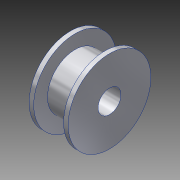
# Autodesk Inventor part: XY_Wheel-SquareBar-Rev3
Saved by Autodesk Inventor 2015 (Build 190159000, 159)
## iProperties
Created: 2017-01-08
Part Number: XY_Wheel-SquareBar-Rev3
Material: Aluminum 6061
Document SubType Name: Modeling
Designer: Guy
Density: 2.7 g/cm^3
Appearance: Aluminum - Flat
Mass: 2.90837 g
Surface Area: 12.4407 cm^2
Volume: 1.07717 cm^3
Author: Guy
Autodesk Inventor part; units mm, degrees
ref_plane "YZ Plane" through (0, 0, 0) normal (1, 0, 0) x (0, 1, 0)
ref_plane "XZ Plane" through (0, 0, 0) normal (0, 1, 0) x (-1, 0, 0)
ref_plane "XY Plane" through (0, 0, 0) normal (0, 0, 1) x (1, 0, 0)
sketch "Sketch1" plane through (0, 0, 0) normal (0, 0, 1) x (1, 0, 0)
  line L0 (0, 0) -> (0, 9)
  line L1 (0, 9) -> (1, 9)
  line L2 (1, 9) -> (1, 6)
  line L3 (1, 6) -> (7.5, 6)
  line L4 (7.5, 6) -> (7.5, 9)
  line L5 (7.5, 9) -> (8.5, 9)
  line L6 (8.5, 9) -> (8.5, 0)
  line L7 (8.5, 0) -> (0, 0)
  dimension "d0" = 8.5
  dimension "d1" = 9
  dimension "d2" = 6.5
  dimension "d3" = 6
  dimension "d9" = 1
  constraints: 16 end point, 6 perpendicular, 2 point on line, 1 vertical
  measures "d0" distance between parallel lines of L0 L6
  measures "d1" distance between parallel lines of L7 L1
  measures "d2" distance between parallel lines of L2 L4
  measures "d3" distance between parallel lines of L7 L3
  measures "d9" distance between parallel lines of L0 L2
revolve "Revolution1" add sketch "Sketch1" angle 360 about axis through (8.5, 0, 0) along (-1, 0, 0)
sketch "Sketch2" plane through (8.5, 0, 0) normal (1, 0, 0) x (0, 0, -1)
  circle A0 centre (0, 0) radius 9 projected
  circle A1 centre (0, 0) radius 2.5
  dimension "d6" = 5
  constraints: 1 centre point, 1 coincident
  measures "d6" diameter of A1
extrude "Extrusion1" cut sketch "Sketch2" against normal up to next contours A1
body "Solid1"
